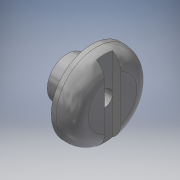
# Autodesk Inventor part: nutsert
Saved by Autodesk Inventor 2019 (Build 230136000, 136)
## iProperties
Created: 2020-03-06
Part Number: nutsert
Material: Generic
Document SubType Name: Modeling
Designer: ntb11189
Density: 1 g/cm^3
Appearance: Steel
Author: ntb11189
Autodesk Inventor part; units mm, degrees
ref_plane "YZ Plane" through (0, 0, 0) normal (1, 0, 0) x (0, 1, 0)
ref_plane "XZ Plane" through (0, 0, 0) normal (0, 1, 0) x (-1, 0, 0)
ref_plane "XY Plane" through (0, 0, 0) normal (0, 0, 1) x (1, 0, 0)
sketch "Sketch1" plane through (0, 0, 0) normal (1, 0, 0) x (0, 1, 0)
  circle A0 centre (0, 0) radius 5
  dimension "d0" = 5
  constraints: 1 centre point, 1 coincident
  measures "d0" radius of A0
extrude "Extrusion1" add sketch "Sketch1" along normal blind 2.6
fillet "Fillet1" radius 2 1 edges at (2.6, -5, 0)
sketch "Sketch2" plane through (2.6, 0, 0) normal (1, 0, 0) x (0, 0, -1)
  circle A0 centre (0, 0) radius 3 projected
  circle A1 centre (0, 0) radius 5 projected
  circle A2 centre (0, 0) radius 3 projected
  circle A3 centre (0, 0) radius 5 projected
  line L0 (1, 4.899) -> (1, -4.899)
  line L1 (-1, 4.899) -> (-1, -4.899)
  dimension "d4" = 1
  dimension "d5" = 1
  constraints: 4 end point, 4 point on circle, 1 parallel, 1 vertical
  measures "d4" distance from line of point (0, 0) L1
  measures "d5" distance from line of L0 point (0, 0)
extrude "Extrusion2" cut sketch "Sketch2" against normal blind 1 contours L0 A0 L1 | A0 L1 A1 L0 | L0 A1 L1 A0
sketch "Sketch3" plane through (0, 0, 0) normal (-1, 0, 0) x (0, 0, 1)
  circle A0 centre (0, 0) radius 2.5
  dimension "d8" = 2.5
  constraints: 1 centre point, 1 coincident
  measures "d8" radius of A0
extrude "Extrusion3" add sketch "Sketch3" along normal blind 3
sketch "Sketch4" plane through (-3, 0, 0) normal (-1, 0, 0) x (0, 0, 1)
  circle A0 centre (0, 0) radius 1
  dimension "d11" = 1
  constraints: 1 centre point, 1 coincident
  measures "d11" radius of A0
extrude "Extrusion4" cut sketch "Sketch4" against normal through all
body "Solid1"
